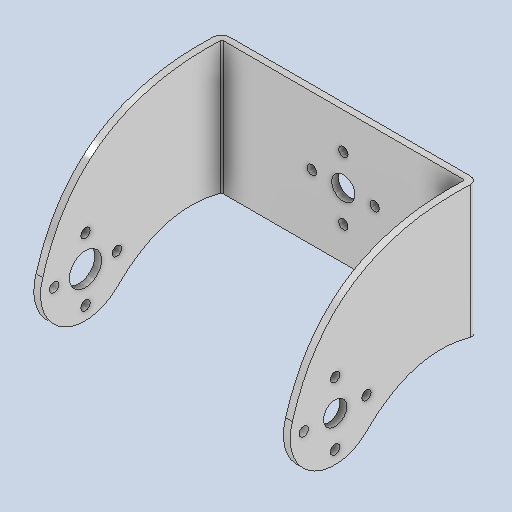
# Autodesk Inventor part: axis_15_bottom_frame
Saved by Autodesk Inventor 2026.1 (Build 301233020, 233B)
## iProperties
Created: 2023-10-27
Part Number: axis_15_bottom_frame
Material: Aluminum 6061-AHC
Document SubType Name: Sheet Metal
Designer: chanh
Density: 2.7 g/cm^3
Sheet Metal Rule: Default_mm
Appearance: Aluminum - Dark
Author: chanh
Autodesk Inventor part; units mm, degrees
ref_plane "YZ Plane" through (0, 0, 0) normal (1, 0, 0) x (0, 1, 0)
ref_plane "XZ Plane" through (0, 0, 0) normal (0, 1, 0) x (-1, 0, 0)
ref_plane "XY Plane" through (0, 0, 0) normal (0, 0, 1) x (1, 0, 0)
sketch "Sketch1" plane through (0, 0, 0) normal (0, 0, 1) x (1, 0, 0)
  line L0 (-28.59, -25) -> (28.59, -25)
  line L1 (28.59, -25) -> (28.59, 25)
  line L2 (28.59, 25) -> (-28.59, 25)
  line L3 (-28.59, 25) -> (-28.59, -25)
  line L4 (-28.59, -25) -> (28.59, 25) construction
  line L5 (28.59, -25) -> (-28.59, 25) construction
  point P0 (0, 0)
  dimension "d0" = 57.18
  dimension "d1" = 50
  measures "d0" distance of L2.end L1.end
  measures "d1" distance of L1.end L0.end
extrude "Plate1" add sketch "Sketch1" along normal blind 1.5
sketch "Sketch2" plane through (-27.09, -25, 0) normal (-1, 0, 0) x (0, -1, 0)
  line L0 (-50, 0) -> (0, 0)
  line L1 (0, 0) -> (0, 45)
  line L2 (0, 45) -> (-50, 45)
  line L3 (-50, 45) -> (-50, 0)
  constraints: 6 end point, 1 horizontal, 1 perpendicular, 1 vertical
edge flange "Flange1" height 45 angle 90 thickness 1.5 bend radius 0.31 thickness toward (-1, 0, 0) relief tear relief width 1.5 relief depth 0.75 corner gap 0.31 corner form 0 edges at (-28.59, 0, 1.5) (28.59, 0, 1.5) wall of the first edge with corners at (-27.09, 25, 0) (-27.09, -25, 0) (-27.09, -25, 45) (-27.09, 25, 45)
bend "Bend1"
corner "Corner1"
sketch "Sketch17" plane through (0, 0, 1.5) normal (0, 0, 1) x (1, 0, 0)
  circle A0 centre (0, 7) radius 0.7835
  circle A1 centre (7, 0) radius 0.7835
  circle A2 centre (0, -7) radius 0.7835
  circle A3 centre (-7, 0) radius 0.7835
  point P0 (0, 0)
  constraints: 4 centre point, 8 other
hole "Hole7" at (0, 7, 1.5) at (7, 0, 1.5) at (0, -7, 1.5) at (-7, 0, 1.5) direction (0, 0, -1) diameter 2.1 depth 1.5
sketch "Sketch26" plane through (28.59, -25, 45) normal (1, 0, 0) x (0, 0, -1)
  arc A0 (3.5502, 14.1468) -> (20.0473, 3.9617) centre (13, 11) ccw
  line L0 (45, 50) -> (45, 0) projected
  spline S0 degree 2 poles (3.5502, 14.1468) (11.7245, 42.1837) (45, 40) knots 0 0 0 1 1 1
  spline S1 degree 2 poles (20.0473, 3.9617) (31.1315, 14.9193) (45, 10) knots 0 0 0 1 1 1
  line L1 (45, 10) -> (45, 40)
  line L2 (0, 0) -> (45, 0)
  line L3 (45, 0) -> (45, 50)
  line L4 (45, 50) -> (0, 50)
  line L5 (0, 50) -> (0, 0)
  point P0 (45, 25)
  point P1 (45, 25)
  point P2 (17.1562, 34.0829)
  point P3 (32.0366, 10.9995)
  dimension "d143" = 19.92
  dimension "d144" = 32
  dimension "d145" = 14
  dimension "d160" = 15
  dimension "d161" = 15
  dimension "d162" = 7.0473
  dimension "d163" = 9.4498
  dimension "d164" = 19.0366
  dimension "d165" = 7.0378
  dimension "d166" = 13.606
  dimension "d167" = 19.9361
  constraints: 10 end point, 2 parallel, 2 point on circle, 2 point on line, 1 centre point, 1 collinear, 1 horizontal, 1 midpoint, 1 perpendicular, 8 other
  measures "d143" diameter of A0
  measures "d144" horizontal distance of point (45, 25) A0.centre
  measures "d145" vertical distance of point (45, 25) A0.centre
  measures "d160" distance of point (45, 25) L1.end
  measures "d161" distance of point (45, 25) L1.start
  measures "d162" horizontal distance of A0.centre A0.end
  measures "d163" horizontal distance of A0.centre A0.start
  measures "d164" distance of A0.centre point (32.037, 11)
  measures "d165" vertical distance of A0.end point (32.037, 11)
  measures "d166" horizontal distance of point (17.156, 34.083) A0.start
  measures "d167" vertical distance of point (17.156, 34.083) A0.start
extrude "Cut8" cut sketch "Sketch26" against normal blind 57.18 contours A0 S1 L0 L2 L5 L4 S0
sketch "Sketch27" plane through (-28.59, -14.4222, 1.81) normal (-1, 0, 0) x (0, 0, 1)
  circle A0 centre (23.12, 0.4222) radius 0.7835 projected
  circle A1 centre (30.12, -6.5778) radius 0.7835 projected
  circle A2 centre (30.12, 7.4222) radius 0.7835 projected
  circle A3 centre (37.12, 0.4222) radius 0.7835 projected
  point P0 (-1.81, 14.4222)
hole "Hole15" at (-28.59, -14, 24.93) at (-28.59, -7, 31.93) at (-28.59, -21, 31.93) at (-28.59, -14, 38.93) direction (1, 0, 0) diameter 2.1 depth 1.5
sketch "Sketch28" plane through (28.59, -14.4222, 1.81) normal (1, 0, 0) x (0, 0, -1)
  circle A0 centre (-23.12, 0.4222) radius 0.7835 projected
  circle A1 centre (-30.12, -6.5778) radius 0.7835 projected
  circle A2 centre (-37.12, 0.4222) radius 0.7835 projected
  circle A3 centre (-30.12, 7.4222) radius 0.7835 projected
  point P0 (1.81, 14.4222)
hole "Hole16" at (28.59, -14, 24.93) at (28.59, -7, 31.93) at (28.59, -21, 31.93) at (28.59, -14, 38.93) direction (-1, 0, 0) diameter 2.1 depth 1.5
sketch "Sketch29" plane through (-28.59, -14.4222, 1.81) normal (-1, 0, 0) x (0, 0, 1)
  circle A0 centre (30.12, 0.4222) radius 1.2295 projected
  point P0 (-1.81, 14.4222)
hole "Hole17" at (-28.59, -14, 31.93) direction (1, 0, 0) diameter 7.2 depth 1.5
sketch "Sketch30" plane through (28.59, -14.4222, 1.81) normal (1, 0, 0) x (0, 0, -1)
  circle A0 centre (-30.12, 0.4222) radius 1.75 projected
  point P0 (1.81, 14.4222)
hole "Hole18" at (28.59, -14, 31.93) direction (-1, 0, 0) diameter 5.2 depth 1.5
sketch "Sketch31" plane through (0, 0, 1.5) normal (0, 0, 1) x (1, 0, 0)
  circle A0 centre (0, 0) radius 1.75 projected
  point P0 (0, 0)
hole "Hole19" at (0, 0, 1.5) direction (0, 0, -1) diameter 5.2 depth 1.5
equation "\"d90\" = Thickness"
equation "\"d2\" = Thickness"
equation "\"d3\" = BendReliefWidth"
equation "\"d4\" = BendReliefDepth"
equation "\"d5\" = MinimumRemnant"
equation "\"d6\" = TransitionRadius"
equation "\"d9\" = BendRadius"
equation "\"d10\" = CornerReliefSize"
equation "\"d11\" = GapSize"
equation "\"d12\" = JacobiRadiusSize"
equation "\"BendReliefWidth\" = Thickness"
equation "\"BendReliefDepth\" = 0.5 * Thickness"
equation "\"CornerReliefSize\" = 4 * Thickness"
equation "\"MinimumRemnant\" = 2 * Thickness"
equation "\"TransitionRadius\" = BendRadius"
equation "\"JacobiRadiusSize\" = BendRadius"
equation "\"GapSize\" = Thickness"
equation "\"Thickness\" = 1.5"
equation "\"BendRadius\" = 0.31"
body "Solid1"
